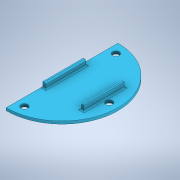
# Autodesk Inventor part: Base1
Saved by Autodesk Inventor 2020 (Build 240168000, 168)
## iProperties
Created: 2020-10-28
Part Number: Base1
Material: PC/ABS Plastic
Document SubType Name: Modeling
Designer: aaron
Density: 0.357273 g/cm^3
Appearance: Turquoise
Author: aaron
Autodesk Inventor part; units mm, degrees
ref_plane "YZ Plane" through (0, 0, 0) normal (1, 0, 0) x (0, 1, 0)
ref_plane "XZ Plane" through (0, 0, 0) normal (0, 1, 0) x (-1, 0, 0)
ref_plane "XY Plane" through (0, 0, 0) normal (0, 0, 1) x (1, 0, 0)
sketch "Sketch1" plane through (0, 0, 0) normal (0, 1, 0) x (-1, 0, 0)
  circle A0 centre (0, 0) radius 41.5 construction
  line L0 (0, -41.5) -> (0, 41.5)
  arc A1 (0, 41.5) -> (0, -41.5) centre (0, 0) ccw
  circle A2 centre (-6, -34) radius 2.5
  circle A3 centre (-6, 34) radius 2.5
  line L1 (0, 0) -> (-41.5, 0) construction
  circle A4 centre (-35, 0) radius 2.5
  dimension "d0" = 83
  dimension "d1" = 83
  dimension "d2" = 5
  dimension "d3" = 6
  dimension "d4" = 34
  dimension "d5" = 34
  dimension "d6" = 35
  constraints: 5 centre point, 5 point on circle, 4 end point, 3 equal radius, 1 coincident, 1 point on line, 1 vertical, 1 vertical alignment
  measures "d0" diameter of A0
  measures "d1" distance of L0.start L0.end
  measures "d2" diameter of A2
  measures "d3" horizontal distance of point (0, 0) A2.centre
  measures "d4" vertical distance of point (0, 0) A2.centre
  measures "d5" vertical distance of point (0, 0) A3.centre
  measures "d6" distance of point (0, 0) A4.centre
extrude "Extrusion1" add sketch "Sketch1" along normal blind 2
sketch "Espacio9V" plane through (0, 2, 0) normal (0, 1, 0) x (1, 0, 0)
  line L0 (2.75, -24.25) -> (29.25, -24.25)
  line L1 (29.25, -24.25) -> (29.25, 24.25)
  line L2 (29.25, 24.25) -> (2.75, 24.25)
  line L3 (2.75, 24.25) -> (2.75, -24.25)
  line L4 (2.75, -24.25) -> (29.25, 24.25) construction
  line L5 (29.25, -24.25) -> (2.75, 24.25) construction
  line L6 (0, 0) -> (41.5, 0) construction
  arc A0 (0, -41.5) -> (0, 41.5) centre (0, 0) ccw construction
  point P0 (16, 0)
  dimension "d11" = 26.5
  dimension "d12" = 48.5
  dimension "d13" = 16
  constraints: 14 end point, 2 horizontal, 2 midpoint, 2 parallel, 1 perpendicular, 1 point on circle, 1 point on line
  measures "d11" distance of L1.end L2.end
  measures "d12" distance of L2.end L0.start
  measures "d13" distance of point (16, 0) L6.start
sketch "Sketch3" plane through (0, 0, 0) normal (0, 0, 1) x (1, 0, 0)
  line L0 (29.25, 2) -> (31.25, 2)
  line L1 (31.25, 2) -> (31.25, 6)
  line L2 (31.25, 6) -> (29.25, 6)
  line L3 (29.25, 6) -> (29.25, 2)
  line L4 (2.75, 2) -> (0.75, 2)
  line L5 (0.75, 2) -> (0.75, 6)
  line L6 (0.75, 6) -> (2.75, 6)
  line L7 (2.75, 6) -> (2.75, 2)
  point P0 (0, 0)
  point P1 (2.75, 2)
  dimension "d14" = 2
  dimension "d15" = 4
  dimension "d16" = 4
  dimension "d17" = 2
  constraints: 16 end point, 4 parallel, 2 horizontal, 2 perpendicular
  measures "d14" distance of L0.start L0.end
  measures "d15" distance of L0.end L1.end
  measures "d16" distance of L4.end L5.end
  measures "d17" distance of L4.start L4.end
extrude "Extrusion2" add sketch "Sketch3" along normal mid plane 30
fillet "Fillet1" radius 1 8 edges at (30.25, 2, 15) (29.25, 2, 0) (30.25, 2, -15) (31.25, 2, 0) (2.75, 2, 0) (1.75, 2, 15) (1.75, 2, -15) (0.75, 2, 0)
fillet "Fillet2" radius 1 2 edges at (2.75, 6, 0) (29.25, 6, 0)
body "Solid1"
